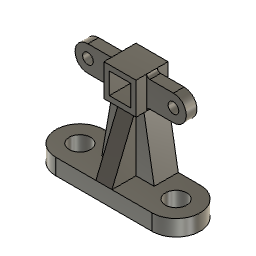
A2_AI22BTECH11005_1 (Autodesk Fusion 360 design; units mm, degrees)
Autodesk Fusion 360 part; units mm, degrees
sketch "Sketch1" plane through (0, 0, 0) normal (0, 1, 0) x (1, 0, 0)
  line L0 (-10, -10) -> (10, -10)
  line L1 (10, -10) -> (10, 10)
  line L2 (10, 10) -> (-10, 10)
  line L3 (-10, 10) -> (-10, -10)
  line L4 (0, 15) -> (15, 15)
  line L5 (15, -15) -> (-15, -15)
  line L6 (0, 15) -> (-15, 15)
  line L7 (0, -15) -> (15, -15)
  line L8 (0, -15) -> (-15, -15)
  line L9 (-15, 15) -> (15, 15)
  line L10 (-40, -12) -> (-18, -12)
  line L11 (-40, 12) -> (-18, 12)
  line L12 (40, 12) -> (18, 12)
  line L13 (40, -12) -> (18, -12)
  arc A0 (-40, 12) -> (-40, -12) centre (-40, 0) ccw
  line L14 (15, 15) -> (15, 15)
  line L15 (15, -15) -> (15, -15)
  arc A1 (40, -12) -> (40, 12) centre (40, 0) ccw
  line L16 (-15, -15) -> (-15, -15)
  line L17 (-15, 15) -> (-15, 15)
  circle A2 centre (-40, 0) radius 5
  circle A3 centre (40, 0) radius 5
  arc A4 (-18, 12) -> (-15, 15) centre (-18, 15) ccw
  arc A5 (15, 15) -> (18, 12) centre (18, 15) ccw
  arc A6 (18, -12) -> (15, -15) centre (18, -15) ccw
  arc A7 (-15, -15) -> (-18, -12) centre (-18, -15) ccw
  line L18 (-15, -15) -> (-15, 15)
  line L19 (15, 15) -> (15, -15)
  line L20 (52, 0) -> (52, 70) construction
  line L21 (-52, 0) -> (-52, 70) construction
  line L22 (0, 70) -> (-24.5, 70)
  line L23 (0, 70) -> (24.5, 70)
  line L24 (-15, 15) -> (-24.5, 70)
  line L25 (15, 15) -> (24.5, 70)
  dimension "d2" = 15
  dimension "d4" = 30
  dimension "d12" = 3
  dimension "d13" = 3
  dimension "d14" = 3
  dimension "d15" = 3
  dimension "d17" = 70
  dimension "d19" = 70
  dimension "d20" = 24.5
  dimension "d21" = 24.5
  constraint horizontal L0
  constraint perpendicular L0 L1
  constraint perpendicular L1 L2
  constraint perpendicular L0 L3
  constraint midpoint L5 L7.start
  constraint parallel L5 L8
  constraint tangent L11 A0
  constraint tangent L12 A1
  constraint tangent L13 A1
  constraint concentric A0 A2
  constraint concentric A1 A3
  constraint tangent L11 A4
  constraint tangent L12 A5
  constraint tangent L13 A6
  constraint tangent L10 A7
  constraint tangent A4 L18
  constraint tangent A6 L19
  constraint midpoint A1 L20.start
  constraint tangent A1 L20
  constraint vertical L20
  constraint midpoint A0 L21.start
  constraint vertical L21
  measures "d2" distance of L4.start L4.end
  measures "d4" distance of L5.start L5.end
  measures "d12" radius of A4
  measures "d13" radius of A5
  measures "d14" radius of A6
  measures "d15" radius of A7
  measures "d17" distance of L20.start L20.end
  measures "d19" distance of L21.start L21.end
  measures "d20" distance of L22.start L22.end
  measures "d21" distance of L22.start L23.end
extrude "Extrude1" add sketch "Sketch1" along normal blind 15 and the other way blind 15 contours L4 L5 L6 L7 L8 L9 L18 L19
extrude "Extrude3" add sketch "Sketch1" along normal blind 5 contours L10 L11 A0 A4 A7 L18
extrude "Extrude4" add sketch "Sketch1" along normal blind 0 and the other way blind 5 contours L10 L11 A0 A4 A7 L18
extrude "Extrude5" add sketch "Sketch1" along normal blind 5 and the other way blind 5 contours L12 L13 A1 A5 A6 L19
extrude "Extrude6" add sketch "Sketch1" along normal blind 15 and the other way blind 7.5 contours L4 L6 L9 L22 L23 L24 L25
sketch "Sketch2" plane through (0, 0, 0) normal (1, 0, 0) x (0, 1, 0)
  line L0 (0, -15) -> (-7.5, -15)
  line L1 (-7.5, -15) -> (-7.5, -70)
  line L2 (-7.5, -70) -> (-30, -70)
  line L3 (-7.5, -15) -> (-30, -70)
  dimension "d44" = 7.5
  dimension "d45" = 22.5
  constraint horizontal L0
  constraint perpendicular L0 L1
  constraint perpendicular L1 L2
  measures "d44" distance of L0.start L0.end
  measures "d45" distance of L1.end L2.end
extrude "Extrude7" add sketch "Sketch2" along normal blind 7.5 and the other way blind 7.5
sketch "Sketch3" plane through (0, 0, -70) normal (0, 0, -1) x (1, 0, 0)
  line L0 (-24.5, 7.5) -> (-24.5, -15)
  line L1 (-24.5, -15) -> (24.5, -15)
  line L2 (24.5, -15) -> (24.5, 7.5)
  line L3 (24.5, 7.5) -> (7.5, 7.5)
  line L4 (7.5, 7.5) -> (7.5, 30)
  line L5 (7.5, 30) -> (-7.5, 30)
  line L6 (-7.5, 30) -> (-7.5, 7.5)
  line L7 (-7.5, 7.5) -> (-24.5, 7.5)
  line L8 (0, -15) -> (45, -15)
  line L9 (45, -15) -> (-45, -15)
  line L10 (-45, 30) -> (45, 30)
  arc A0 (-45, -2.5) -> (-45, 17.5) centre (-45, 7.5) ccw
  arc A1 (-45, 17.5) -> (-45, -2.5) centre (-45, 7.5) ccw
  arc A2 (45, -2.5) -> (45, 17.5) centre (45, 7.5) ccw
  arc A3 (45, 17.5) -> (45, -2.5) centre (45, 7.5) ccw
  arc A4 (45, -15) -> (45, 30) centre (45, 7.5) ccw
  arc A5 (-45, 30) -> (-45, -15) centre (-45, 7.5) ccw
  line L11 (-24.5, -15) -> (24.5, -15)
  dimension "d51" = 22.5
  dimension "d52" = 20
  dimension "d53" = 20
  constraint midpoint L1 L8.start
  constraint parallel L1 L8
  constraint perpendicular L0 L9
  constraint perpendicular L4 L10
  constraint concentric A0 A1
  constraint concentric A2 A3
  constraint coincident L0.end L1.start
  constraint coincident L1.end L2.start
  measures "d51" distance of L10.start A0.centre
  measures "d52" diameter of A0
  measures "d53" diameter of A2
extrude "Extrude8" add sketch "Sketch3" along normal blind 15
extrude "Extrude2" [suppressed]
